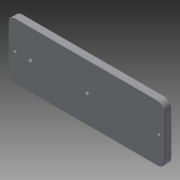
# Autodesk Inventor part: BasePlateTL
Saved by Autodesk Inventor 2015 (Build 190159000, 159)
## iProperties
Created: 2015-02-09
Part Number: BasePlateTL
Material: Generic
Document SubType Name: Modeling
Designer: PLTW-Stu-02
Density: 1 g/cm^3
Appearance: Default
Author: PLTW-Stu-02
Autodesk Inventor part; units mm, degrees
ref_plane "YZ Plane" through (0, 0, 0) normal (1, 0, 0) x (0, 1, 0)
ref_plane "XZ Plane" through (0, 0, 0) normal (0, 1, 0) x (-1, 0, 0)
ref_plane "XY Plane" through (0, 0, 0) normal (0, 0, 1) x (1, 0, 0)
sketch "Sketch1" plane through (0, 0, 0) normal (0, 0, 1) x (1, 0, 0)
  line L0 (22.1008, 26.4872) -> (276.1008, 26.4872)
  line L1 (288.8008, 13.7872) -> (288.8008, -62.4128)
  line L2 (276.1008, -75.1128) -> (22.1008, -75.1128)
  line L3 (9.4008, -62.4128) -> (9.4008, 13.7872)
  arc A0 (12.5758, 26.4872) -> (9.4008, 23.3122) centre (12.5758, 23.3122) ccw
  arc A1 (22.1008, 26.4872) -> (9.4008, 13.7872) centre (22.1008, 13.7872) ccw
  arc A2 (9.4008, -62.4128) -> (22.1008, -75.1128) centre (22.1008, -62.4128) ccw
  arc A3 (276.1008, -75.1128) -> (288.8008, -62.4128) centre (276.1008, -62.4128) ccw
  arc A4 (288.8008, 13.7872) -> (276.1008, 26.4872) centre (276.1008, 13.7872) ccw
  point P0 (0, 0)
  point P1 (288.8008, -75.1128)
  point P2 (288.8008, 26.4872)
  point P3 (9.4008, -75.1128)
  point P4 (20.5133, -24.3128)
  point P5 (47.5008, -24.3128)
  point P6 (149.1008, -24.3128)
  point P7 (277.6883, -24.3128)
  dimension "d0" = 279.4
  dimension "d1" = 101.6
  dimension "d3" = 12.7
  dimension "d41" = 11.1125
  dimension "d42" = 11.1125
  constraints: 10 point on circle, 10 tangent, 8 end point, 8 point on line, 5 centre point, 3 equal radius, 2 parallel, 1 horizontal, 1 perpendicular
  measures "d0" distance of point (288.801, -75.113) point (9.401, -75.113)
  measures "d1" distance of point (288.801, 26.487) point (288.801, -75.113)
  measures "d3" radius of A1
  measures "d41" distance from line of L3 point (20.513, -24.313)
  measures "d42" distance from line of L1 point (277.688, -24.313)
extrude "Extrusion1" add sketch "Sketch1" along normal blind 12.7
chamfer "Chamfer1" distance 0.7937 angle 45 16 edges at (149.1008, 26.4872, 12.7) (13.1205, 22.7675, 12.7) (9.4008, -24.3128, 12.7) (13.1205, -71.3931, 12.7) (149.1008, -75.1128, 12.7) (285.081, -71.3931, 12.7) (288.8008, -24.3128, 12.7) (285.081, 22.7675, 12.7) (149.1008, 26.4872, 0) (13.1205, 22.7675, 0) (9.4008, -24.3128, 0) (13.1205, -71.3931, 0) (149.1008, -75.1128, 0) (285.081, -71.3931, 0) (288.8008, -24.3128, 0) (285.081, 22.7675, 0)
hole "Hole5" at (20.5133, -24.3128, 0) direction (0, 0, 1) diameter 6.35 end through all countersink diameter 12.7 countersink angle 82
hole "Hole6" at (277.6883, -24.3128, 0) direction (0, 0, 1) diameter 6.35 end through all countersink diameter 12.7 countersink angle 82
hole "Hole7" at (47.5008, -24.3128, 0) at (149.1008, -24.3128, 0) direction (0, 0, 1) diameter 7.9375 end through all
sketch "Sketch2" plane through (0, 0, 0) normal (0, 0, -1) x (-1, 0, 0)
  point P0 (0, 0)
  point P1 (-20.5133, 16.4404)
  point P2 (-20.5133, -62.4734)
  point P3 (-277.2648, -62.4734)
  point P4 (-277.2648, 16.4404)
hole "Hole8" at (20.5133, 16.4404, 0) at (20.5133, -62.4734, 0) at (277.2648, -62.4734, 0) at (277.2648, 16.4404, 0) direction (0, 0, 1) diameter 3.302 depth 7.3025 tip angle 118 thread size "8-32 UNC" class "2B" standard "ANSI Unified Screw Threads"
body "Solid1"
